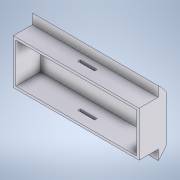
# Autodesk Inventor part: bateria_mocowanie_ramie_robota
Saved by Autodesk Inventor 2021 (Build 250183000, 183)
## iProperties
Created: 2022-01-29
Part Number: bateria_mocowanie_ramie_robota
Material: Generic
Document SubType Name: Modeling
Designer: Łukasz
Density: 1 g/cm^3
Appearance: Opal
Author: Łukasz
Autodesk Inventor part; units mm, degrees
ref_plane "YZ Plane" through (0, 0, 0) normal (1, 0, 0) x (0, 1, 0)
ref_plane "XZ Plane" through (0, 0, 0) normal (0, 1, 0) x (-1, 0, 0)
ref_plane "XY Plane" through (0, 0, 0) normal (0, 0, 1) x (1, 0, 0)
sketch "Sketch1" plane through (0, 0, 0) normal (0, 0, 1) x (1, 0, 0)
  line L0 (0, 0) -> (-151, 0)
  line L1 (-151, 0) -> (-151, 112)
  line L2 (-151, 112) -> (0, 112)
  line L3 (0, 112) -> (0, 0)
  line L4 (-151, 0) -> (0, 0)
  line L5 (0, 0) -> (0, -1)
  line L6 (0, -1) -> (-151, -1)
  line L7 (-151, -1) -> (-151, 0)
  dimension "d0" = 151
  dimension "d1" = 112
  dimension "d35" = 1
  constraints: 16 end point, 4 parallel, 2 horizontal, 2 perpendicular
  measures "d0" distance of L1.end L2.end
  measures "d1" distance of L0.end L1.end
  measures "d35" distance of L4.end L5.end
extrude "Extrusion1" add sketch "Sketch1" along normal blind 3
sketch "Sketch2" plane through (0, 0, 3) normal (0, 0, 1) x (1, 0, 0)
  line L0 (-151, 0) -> (0, 0) projected
  line L1 (0, 0) -> (-151, 0)
  line L2 (-151, 0) -> (-151, 53)
  line L3 (-151, 53) -> (0, 53)
  line L4 (0, 53) -> (0, 0)
  line L5 (-148, 50) -> (-3, 50)
  line L6 (-3, 50) -> (-3, 3)
  line L7 (-3, 3) -> (-148, 3)
  line L8 (-148, 3) -> (-148, 50)
  line L9 (-151, -1) -> (0, -1) projected
  line L10 (-151, 112) -> (-151, -1) projected
  line L11 (0, -1) -> (0, 112) projected
  line L12 (-148, 3) -> (-3, 3)
  line L13 (-3, 3) -> (-3, 2)
  line L14 (-3, 2) -> (-148, 2)
  line L15 (-148, 2) -> (-148, 3)
  dimension "d4" = 151
  dimension "d5" = 53
  dimension "d6" = 3
  dimension "d7" = 3
  dimension "d8" = 3
  dimension "d9" = 3
  dimension "d36" = 1
  constraints: 24 end point, 6 parallel, 3 horizontal, 3 perpendicular, 1 point on line
  measures "d4" distance of L2.end L3.end
  measures "d5" distance of L1.end L2.end
  measures "d6" distance between parallel lines of L3 L5
  measures "d7" distance between parallel lines of L0 L7
  measures "d8" distance between parallel lines of L2 L8
  measures "d9" distance between parallel lines of L4 L6
  measures "d36" distance of L12.end L13.end
extrude "Extrusion2" add sketch "Sketch2" along normal blind 30
sketch "Sketch3" plane through (0, 0, 3) normal (0, 0, 1) x (1, 0, 0)
  line L0 (-148, 109) -> (-103.5, 109)
  line L1 (-103.5, 109) -> (-103.5, 56)
  line L2 (-103.5, 56) -> (-148, 56)
  line L3 (-148, 56) -> (-148, 109)
  line L4 (-47.5, 109) -> (-3, 109)
  line L5 (-3, 109) -> (-3, 56)
  line L6 (-3, 56) -> (-47.5, 56)
  line L7 (-47.5, 56) -> (-47.5, 109)
  line L8 (0, 112) -> (-151, 112) projected
  line L9 (-151, 112) -> (-151, 53) projected
  line L10 (0, 53) -> (0, 112) projected
  line L11 (-85.5, 100) -> (-65.5, 100)
  line L12 (-65.5, 100) -> (-65.5, 65)
  line L13 (-65.5, 65) -> (-85.5, 65)
  line L14 (-85.5, 65) -> (-85.5, 100)
  line L15 (-62.5, 103) -> (-88.5, 103)
  line L16 (-88.5, 103) -> (-88.5, 62)
  line L17 (-88.5, 62) -> (-62.5, 62)
  line L18 (-62.5, 62) -> (-62.5, 103)
  line L19 (-100.5, 112) -> (-151, 112)
  line L20 (-151, 112) -> (-151, 53)
  line L21 (-151, 53) -> (-100.5, 53)
  line L22 (-100.5, 53) -> (-100.5, 112)
  line L23 (0, 112) -> (-50.5, 112)
  line L24 (-50.5, 112) -> (-50.5, 53)
  line L25 (-50.5, 53) -> (0, 53)
  line L26 (0, 53) -> (0, 112)
  point P0 (0, 0)
  dimension "d12" = 44.5
  dimension "d13" = 53
  dimension "d14" = 44.5
  dimension "d15" = 53
  dimension "d16" = 3
  dimension "d17" = 3
  dimension "d18" = 3
  dimension "d19" = 20
  dimension "d20" = 35
  dimension "d21" = 12
  dimension "d22" = 18
  dimension "d23" = 3
  dimension "d24" = 3
  dimension "d25" = 3
  constraints: 48 end point, 12 parallel, 6 perpendicular, 3 horizontal, 1 point on line, 9 other
  measures "d12" distance of L1.end L2.end
  measures "d13" distance of L0.end L1.end
  measures "d14" distance of L5.end L6.end
  measures "d15" distance of L4.end L5.end
  measures "d16" distance between parallel lines of L8 L0
  measures "d17" distance between parallel lines of L9 L3
  measures "d18" distance between parallel lines of L5 L10
  measures "d19" distance of L12.end L13.end
  measures "d20" distance of L11.end L12.end
  measures "d21" distance between parallel lines of L8 L11
  measures "d22" distance between parallel lines of L7 L12
  measures "d23" distance between parallel lines of L11 L15
  measures "d24" distance between parallel lines of L0 L19
  measures "d25" distance between parallel lines of L4 L23
extrude "Extrusion3" add sketch "Sketch3" along normal blind 8
fillet "Fillet1" radius 4 6 edges at (-100.5, 82.5, 3) (-62.5, 82.5, 3) (-50.5, 82.5, 3) (-75.5, 103, 3) (-88.5, 82.5, 3) (-75.5, 62, 3)
sketch "Sketch6" plane through (-151, -1, 0) normal (0, -1, 0) x (1, 0, 0)
  line L0 (65.5, 21) -> (85.5, 21)
  line L1 (85.5, 21) -> (85.5, 18)
  line L2 (85.5, 18) -> (65.5, 18)
  line L3 (65.5, 18) -> (65.5, 21)
  line L4 (0, 0) -> (0, 33) projected
  line L5 (0, 33) -> (151, 33) projected
  point P0 (151, 0)
  dimension "d37" = 20
  dimension "d38" = 3
  dimension "d39" = 65.5
  dimension "d40" = 12
  constraints: 8 end point, 2 parallel, 1 horizontal, 1 perpendicular
  measures "d37" distance of L1.end L2.end
  measures "d38" distance of L0.end L1.end
  measures "d39" distance between parallel lines of L4 L3
  measures "d40" distance between parallel lines of L5 L0
extrude "Extrusion5" cut sketch "Sketch6" against normal up to surface (54 mm away)
sketch "Sketch7" plane through (0, 0, 11) normal (0, 0, 1) x (1, 0, 0)
  line L0 (0, 112) -> (-151, 112) projected
  line L1 (0, 112) -> (-151, 112)
  line L2 (-151, 112) -> (-151, 53)
  line L3 (-151, 53) -> (0, 53)
  line L4 (0, 53) -> (0, 112)
  point P0 (0, 0)
  constraints: 8 end point, 2 parallel, 1 horizontal, 1 perpendicular
extrude "Extrusion6" cut sketch "Sketch7" against normal up to surface (11 mm away)
sketch "Sketch8" plane through (-151, -1, 0) normal (-1, 0, 0) x (0, 0, 1)
  arc A0 (38.3305, 78.7131) -> (30.8341, -23.2131) centre (44.5445, 27.0173) ccw
  line L0 (10, 65.9756) -> (10, -11.9409)
  line L1 (10, 65.9756) -> (87.9165, 65.9756) construction
  line L2 (0, 54) -> (33, 54) projected
  line L3 (0, 0) -> (33, 0) projected
  point P0 (0, 1)
  point P1 (0.0136, 54)
  point P2 (10, 54)
  point P3 (10, 0)
  point P4 (0.0346, 0)
  dimension "d45" = 90
  constraints: 4 end point, 4 point on circle, 1 centre point, 1 horizontal, 1 perpendicular
  measures "d45" angle of L0 L1
extrude "Extrusion7" add sketch "Sketch8" against normal up to surface (151 mm away) contours L0 L2 A0 | L3 L0 A0
body "Solid1"
